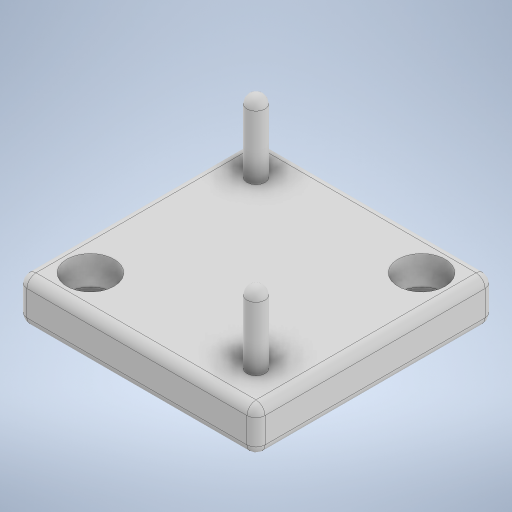
# Autodesk Inventor part: pigeon Mount
Saved by Autodesk Inventor 2023.2 (Build 272271000, 271)
## iProperties
Created: 2023-03-06
Part Number: pigeon Mount
Material: Generic
Document SubType Name: Modeling
Designer: matth
Density: 1 g/cm^3
Appearance: Default
Author: matth
Autodesk Inventor part; units mm, degrees
ref_plane "YZ Plane" through (0, 0, 0) normal (1, 0, 0) x (0, 1, 0)
ref_plane "XZ Plane" through (0, 0, 0) normal (0, 1, 0) x (-1, 0, 0)
ref_plane "XY Plane" through (0, 0, 0) normal (0, 0, 1) x (1, 0, 0)
sketch "Sketch1" plane through (0, 0, 0) normal (0, 1, 0) x (-1, 0, 0)
  circle A0 centre (19.5118, 57.0521) radius 2.5797
  circle A1 centre (19.5118, 28.0961) radius 1.5875
  circle A2 centre (-9.4442, 28.0961) radius 2.5797
  circle A3 centre (-9.4442, 57.0521) radius 1.5875
  line L0 (25.8618, 63.4021) -> (-15.7942, 63.4021)
  line L1 (-15.7942, 63.4021) -> (-15.7942, 21.7461)
  line L2 (-15.7942, 21.7461) -> (25.8618, 21.7461)
  line L3 (25.8618, 21.7461) -> (25.8618, 63.4021)
  point P0 (0, 0)
  dimension "d0" = 5.1594
  dimension "d1" = 3.175
  dimension "d2" = 28.956
  dimension "d3" = 5.1594
  dimension "d4" = 3.175
  dimension "d5" = 28.956
  dimension "d6" = 28.956
  dimension "d7" = 28.956
  dimension "d8" = 41.656
  dimension "d9" = 41.656
  dimension "d10" = 6.35
  dimension "d11" = 6.35
  constraints: 8 end point, 4 centre point, 2 horizontal alignment, 2 parallel, 1 horizontal, 1 perpendicular
  measures "d0" diameter of A0
  measures "d1" diameter of A1
  measures "d2" distance of A1.centre A0.centre
  measures "d3" diameter of A2
  measures "d4" diameter of A3
  measures "d5" distance of A2.centre A3.centre
  measures "d6" distance of A2.centre A1.centre
  measures "d7" distance of A3.centre A0.centre
  measures "d8" distance of L2.end L1.end
  measures "d9" distance of L1.end L0.end
  measures "d10" distance from line of L3 A0.centre
  measures "d11" distance from line of L0 A0.centre
extrude "Extrusion1" add sketch "Sketch1" along normal blind 7.62
sketch "Sketch2" plane through (0, 7.62, 0) normal (0, 1, 0) x (1, 0, 0)
  circle A0 centre (-19.5118, -57.0521) radius 2.5797 projected
  circle A1 centre (-19.5118, -57.0521) radius 4.1275
  circle A2 centre (9.4442, -28.0961) radius 2.5797 projected
  circle A3 centre (9.4442, -28.0961) radius 4.1275
  point P0 (0, 0)
  dimension "d14" = 8.255
  dimension "d15" = 8.255
  constraints: 2 centre point, 2 coincident
  measures "d14" diameter of A1
  measures "d15" diameter of A3
extrude "Extrusion2" cut sketch "Sketch2" against normal blind 5.08 contours A0 | A1 | A2 | A3
sketch "Sketch3" plane through (0, 0, 0) normal (0, -1, 0) x (1, 0, 0)
  circle A0 centre (-19.5118, 28.0961) radius 1.5875 projected
  circle A1 centre (-19.5118, 28.0961) radius 1.5875
  circle A2 centre (9.4442, 57.0521) radius 1.5875 projected
  circle A3 centre (9.4442, 57.0521) radius 1.5875
  point P0 (0, 0)
  constraints: 2 centre point, 2 coincident
extrude "Extrusion3" add sketch "Sketch3" against normal blind 20.32
fillet "Fillet1" radius 1.5875 8 edges at (-25.8618, 7.62, 42.5741) (-5.0338, 7.62, 21.7461) (15.7942, 7.62, 42.5741) (-5.0338, 7.62, 63.4021) (-5.0338, 0, 63.4021) (-25.8618, 0, 42.5741) (-5.0338, 0, 21.7461) (15.7942, 0, 42.5741)
fillet "Fillet2" radius 1.5875 2 edges at (7.8567, 20.32, 57.0521) (-21.0993, 20.32, 28.0961)
fillet "Fillet3" radius 1.5875 12 edges at (15.3292, 7.155, 62.9372) (15.3292, 0.465, 62.9372) (15.7942, 3.81, 63.4021) (15.3292, 7.155, 22.2111) (15.3292, 0.465, 22.2111) (15.7942, 3.81, 21.7461) (-25.3968, 7.155, 22.2111) (-25.3968, 0.465, 22.2111) (-25.8618, 3.81, 21.7461) (-25.3968, 7.155, 62.9372) (-25.3968, 0.465, 62.9372) (-25.8618, 3.81, 63.4021)
body "Solid1"
